Autodesk Inventor part; units mm, degrees
(part 3 of 3)
  line L415 (-154.8147, -40.8229) -> (-168.8197, -40.8229)
  line L416 (-168.8197, -40.8229) -> (-168.8197, -26.8179)
  line L417 (-168.8197, -26.8179) -> (-154.8147, -40.8229) construction
  line L418 (-154.8147, -26.8179) -> (-168.8197, -40.8229) construction
  line L419 (-187.8697, -26.8179) -> (-173.8647, -26.8179)
  line L420 (-173.8647, -26.8179) -> (-173.8647, -40.8229)
  line L421 (-173.8647, -40.8229) -> (-187.8697, -40.8229)
  line L422 (-187.8697, -40.8229) -> (-187.8697, -26.8179)
  line L423 (-187.8697, -26.8179) -> (-173.8647, -40.8229) construction
  line L424 (-173.8647, -26.8179) -> (-187.8697, -40.8229) construction
  line L425 (-214.0317, -26.8179) -> (-200.0267, -26.8179)
  line L426 (-200.0267, -26.8179) -> (-200.0267, -40.8229)
  line L427 (-200.0267, -40.8229) -> (-214.0317, -40.8229)
  line L428 (-214.0317, -40.8229) -> (-214.0317, -26.8179)
  line L429 (-214.0317, -26.8179) -> (-200.0267, -40.8229) construction
  line L430 (-200.0267, -26.8179) -> (-214.0317, -40.8229) construction
  line L431 (-205.1417, -45.8679) -> (-191.1367, -45.8679)
  line L432 (-191.1367, -45.8679) -> (-191.1367, -59.8729)
  line L433 (-191.1367, -59.8729) -> (-205.1417, -59.8729)
  line L434 (-205.1417, -59.8729) -> (-205.1417, -45.8679)
  line L435 (-205.1417, -45.8679) -> (-191.1367, -59.8729) construction
  line L436 (-191.1367, -45.8679) -> (-205.1417, -59.8729) construction
  line L437 (-181.2657, -45.8679) -> (-167.2607, -45.8679)
  line L438 (-167.2607, -45.8679) -> (-167.2607, -59.8729)
  line L439 (-167.2607, -59.8729) -> (-181.2657, -59.8729)
  line L440 (-181.2657, -59.8729) -> (-181.2657, -45.8679)
  line L441 (-181.2657, -45.8679) -> (-167.2607, -59.8729) construction
  line L442 (-167.2607, -45.8679) -> (-181.2657, -59.8729) construction
  line L443 (-83.7297, -45.8679) -> (-69.7247, -45.8679)
  line L444 (-69.7247, -45.8679) -> (-69.7247, -59.8729)
  line L445 (-69.7247, -59.8729) -> (-83.7297, -59.8729)
  line L446 (-83.7297, -59.8729) -> (-83.7297, -45.8679)
  line L447 (-83.7297, -45.8679) -> (-69.7247, -59.8729) construction
  line L448 (-69.7247, -45.8679) -> (-83.7297, -59.8729) construction
  circle A104 centre (-110, -57.5) radius 3.25
  circle A105 centre (0, -57.5) radius 3.25
  line L449 (-143.4772, -45.8679) -> (-143.4772, -58.2679) construction
  line L450 (-9.9772, -45.8679) -> (-9.9772, -58.2679) construction
  line L451 (-219.7432, 11.2821) -> (-213.7432, 11.2821)
  line L452 (-213.7432, 11.2821) -> (-213.7432, -1.1179)
  line L453 (-213.7432, -1.1179) -> (-219.7432, -1.1179)
  line L454 (-219.7432, -1.1179) -> (-219.7432, 11.2821)
  line L455 (-195.7432, 11.2821) -> (-189.7432, 11.2821)
  line L456 (-189.7432, 11.2821) -> (-189.7432, -1.1179)
  line L457 (-189.7432, -1.1179) -> (-195.7432, -1.1179)
  line L458 (-195.7432, -1.1179) -> (-195.7432, 11.2821)
  line L459 (8.4302, -62.3704) -> (-209.6412, -62.3704)
  line L460 (-209.6412, -62.3704) -> (-209.6412, -43.3204)
  line L461 (-209.6412, -43.3204) -> (-223.6412, -43.3204)
  line L462 (-223.6412, -43.3204) -> (-223.6412, 61.3884)
  line L463 (-223.6412, 61.3884) -> (4.4528, 61.3884)
  line L464 (-93, 44) -> (-50, 44)
  line L465 (-50, 44) -> (-50, 37.5)
  line L466 (-50, 37.5) -> (-93, 37.5)
  line L467 (-93, 37.5) -> (-93, 44)
  point P0 (0, 0)
  point P1 (9.3423, 37.558)
  point P2 (-90.4432, 23.3296)
  point P3 (-166.6432, 23.3296)
  point P4 (-190.5192, -14.7704)
  point P5 (-95.2692, -14.7704)
  point P6 (-28.4732, -33.8424)
  point P7 (-85.6172, -33.8204)
  point P8 (-218.2321, -21.7729)
  point P9 (-218.8577, -21.4574)
  dimension "d186" = 0.2
  dimension "d187" = 0.2
  dimension "d188" = 0.2
  dimension "d189" = 0.2
  dimension "d190" = 0.2
  dimension "d191" = 0.2
  dimension "d192" = 0.2
  dimension "d193" = 0.2
  dimension "d194" = 0.2
  dimension "d195" = 0.2
  dimension "d196" = 0.2
  dimension "d198" = 6
  dimension "d199" = 12.4
  dimension "d200" = 6
  dimension "d201" = 14.005
  dimension "d202" = 14.005
  dimension "d203" = 14.005
  dimension "d204" = 14.005
  dimension "d205" = 14.005
  dimension "d206" = 14.005
  dimension "d207" = 14.005
  dimension "d208" = 14.005
  dimension "d209" = 14.005
  dimension "d210" = 14.005
  dimension "d211" = 14.005
  dimension "d212" = 14.005
  dimension "d213" = 14.005
  dimension "d214" = 14.005
  dimension "d215" = 14.005
  dimension "d216" = 14.005
  dimension "d217" = 14.005
  dimension "d218" = 14.005
  dimension "d219" = 14.005
  dimension "d220" = 14.005
  dimension "d221" = 14.005
  dimension "d222" = 14.005
  dimension "d223" = 14.005
  dimension "d224" = 14.005
  dimension "d225" = 14.005
  dimension "d226" = 14.005
  dimension "d227" = 14.005
  dimension "d228" = 14.005
  dimension "d229" = 14.005
  dimension "d230" = 14.005
  dimension "d231" = 14.005
  dimension "d232" = 14.005
  dimension "d233" = 14.005
  dimension "d234" = 14.005
  dimension "d235" = 14.005
  dimension "d236" = 14.005
  dimension "d237" = 14.005
  dimension "d238" = 14.005
  dimension "d239" = 14.005
  dimension "d240" = 14.005
  dimension "d241" = 14.005
  dimension "d242" = 14.005
  dimension "d243" = 14.005
  dimension "d244" = 14.005
  dimension "d245" = 14.005
  dimension "d246" = 14.005
  dimension "d247" = 14.005
  dimension "d248" = 14.005
  dimension "d249" = 14.005
  dimension "d250" = 14.005
  constraints: 776 end point, 128 parallel, 123 midpoint, 72 perpendicular, 63 horizontal, 12 collinear, 10 point on line, 6 centre point, 6 coincident, 5 equal radius, 1 vertical
  measures "d186" distance between parallel lines of L90 L79
  measures "d187" distance from line of point (9.342, 37.558) L80
  measures "d188" distance between parallel lines of L81 L70
  measures "d189" distance between parallel lines of L82 L71
  measures "d190" distance between parallel lines of L83 L72
  measures "d191" distance between parallel lines of L73 L84
  measures "d192" distance between parallel lines of L85 L74
  measures "d193" distance between parallel lines of L86 L75
  measures "d194" distance between parallel lines of L87 L76
  measures "d195" distance between parallel lines of L88 L77
  measures "d196" distance between parallel lines of L89 L78
  measures "d198" distance of L93.start L93.end
  measures "d199" distance of L95.end L93.start
  measures "d200" distance of L97.start L97.end
  measures "d201" distance of L102.end L103.end
  measures "d202" distance of L101.end L102.end
  measures "d203" distance of L108.end L109.end
  measures "d204" distance of L107.end L108.end
  measures "d205" distance of L114.end L115.end
  measures "d206" distance of L113.end L114.end
  measures "d207" distance of L120.end L121.end
  measures "d208" distance of L119.end L120.end
  measures "d209" distance of L126.end L127.end
  measures "d210" distance of L125.end L126.end
  measures "d211" distance of L132.end L133.end
  measures "d212" distance of L131.end L132.end
  measures "d213" distance of L138.end L139.end
  measures "d214" distance of L137.end L138.end
  measures "d215" distance of L144.end L145.end
  measures "d216" distance of L143.end L144.end
  measures "d217" distance of L150.end L151.end
  measures "d218" distance of L149.end L150.end
  measures "d219" distance of L156.end L157.end
  measures "d220" distance of L155.end L156.end
  measures "d221" distance of L162.end L163.end
  measures "d222" distance of L161.end L162.end
  measures "d223" distance of L168.end L169.end
  measures "d224" distance of L167.end L168.end
  measures "d225" distance of L174.end L175.end
  measures "d226" distance of L173.end L174.end
  measures "d227" distance of L180.end L181.end
  measures "d228" distance of L179.end L180.end
  measures "d229" distance of L186.end L187.end
  measures "d230" distance of L185.end L186.end
  measures "d231" distance of L192.end L193.end
  measures "d232" distance of L191.end L192.end
  measures "d233" distance of L198.end L199.end
  measures "d234" distance of L197.end L198.end
  measures "d235" distance of L204.end L205.end
  measures "d236" distance of L203.end L204.end
  measures "d237" distance of L210.end L211.end
  measures "d238" distance of L209.end L210.end
  measures "d239" distance of L216.end L217.end
  measures "d240" distance of L215.end L216.end
  measures "d241" distance of L222.end L223.end
  measures "d242" distance of L221.end L222.end
  measures "d243" distance of L228.end L229.end
  measures "d244" distance of L227.end L228.end
  measures "d245" distance of L234.end L235.end
  measures "d246" distance of L233.end L234.end
  measures "d247" distance of L240.end L241.end
  measures "d248" distance of L239.end L240.end
  measures "d249" distance of L246.end L247.end
  measures "d250" distance of L245.end L246.end
extrude "Thin Plate" add sketch "Sketch5" along normal blind 0.25
sketch "Sketch7" plane through (0, 0, 0.25) normal (0, 0, 1) x (1, 0, 0)
  line L0 (-76.4012, 61.3884) -> (-76.4012, 42.3884) construction
  line L1 (-76.4012, 42.3884) -> (-194.4012, 42.3884) construction
  line L2 (-93, 44) -> (-50, 44) construction
  line L3 (-93, 37.5) -> (-93, 44) construction
  line L4 (-66.3852, 42.3884) -> (-66.3852, 61.3884) construction
  line L5 (51.6148, 42.3884) -> (-66.3852, 42.3884) construction
  line L6 (-50, 44) -> (-50, 37.5) construction
  line L7 (-204.6412, 61.3884) -> (-204.6412, 42.3884) construction
  line L8 (-204.6412, 42.3884) -> (-223.6412, 42.3884) construction
  line L9 (71.4568, 32.8296) -> (-223.6412, 32.8296) construction
  line L10 (14.2318, 13.9046) -> (14.2318, 37.558) construction
  line L11 (4.4528, 13.9046) -> (14.2318, 13.9046) projected
  line L12 (4.4528, -5.3455) -> (4.4528, 13.9046) projected
  line L13 (9.6598, -5.3455) -> (4.4528, -5.3455) projected
  line L14 (9.6598, -24.1954) -> (9.6598, -5.3455) projected
  line L15 (0.0048, -24.1954) -> (9.6598, -24.1954) projected
  line L16 (0.0048, -49.2614) -> (0.0048, -24.1954) projected
  line L17 (8.4302, -49.2614) -> (0.0048, -49.2614) projected
  line L18 (8.4302, -62.3704) -> (8.4302, -49.2614) projected
  line L19 (-209.6412, -62.3704) -> (8.4302, -62.3704) construction
  line L20 (-209.6412, -43.3204) -> (-209.6412, -62.3704) projected
  line L21 (8.4302, -62.3704) -> (-209.6412, -62.3704)
  line L22 (-223.6412, -43.3204) -> (-209.6412, -43.3204) projected
  line L23 (-223.6412, 61.3884) -> (-223.6412, -43.3204) construction
  line L24 (-223.6412, -43.3204) -> (-223.6412, 32.8296)
  line L25 (-223.6412, 61.3884) -> (-223.6412, -43.3204) projected
  line L26 (-223.6412, 32.8296) -> (14.2318, 32.8296)
  line L27 (14.2318, 32.8296) -> (14.2318, 13.9046)
  line L28 (4.4528, 37.558) -> (4.4528, 61.3884) construction
  line L29 (4.4528, 61.3884) -> (-223.6412, 61.3884) construction
  line L30 (-194.4012, 42.3884) -> (-194.4012, 61.3884) construction
  line L31 (-223.6412, 42.3884) -> (-223.6412, 61.3884)
  line L32 (-223.6412, 61.3884) -> (-204.6412, 61.3884)
  line L33 (-204.6412, 61.3884) -> (-204.6412, 42.3884)
  line L34 (-204.6412, 42.3884) -> (-223.6412, 42.3884)
  line L35 (-194.4012, 42.3884) -> (-194.4012, 61.3884)
  line L36 (-194.4012, 61.3884) -> (-76.4012, 61.3884)
  line L37 (-76.4012, 61.3884) -> (-76.4012, 44)
  line L38 (-76.4012, 44) -> (-93, 44)
  line L39 (-93, 44) -> (-93, 42.3884)
  line L40 (-93, 37.5) -> (-93, 44) projected
  line L41 (-93, 42.3884) -> (-194.4012, 42.3884)
  line L42 (-66.3852, 61.3884) -> (-66.3852, 44)
  line L43 (-66.3852, 44) -> (-50, 44)
  line L44 (-50, 44) -> (-50, 42.3884)
  line L45 (-50, 42.3884) -> (4.4528, 42.3884)
  line L46 (4.4528, 42.3884) -> (4.4528, 61.3884)
  line L47 (4.4528, 61.3884) -> (-66.3852, 61.3884)
  line L48 (0.0048, -49.2614) -> (0.0048, -24.1954) projected
  line L49 (0.0048, -24.1954) -> (9.6598, -24.1954) projected
  line L50 (9.6598, -24.1954) -> (9.6598, -5.3455) projected
  line L51 (9.6598, -5.3455) -> (4.4528, -5.3455) projected
  line L52 (4.4528, -5.3455) -> (4.4528, 13.9046) projected
  line L53 (4.4528, 13.9046) -> (14.2318, 13.9046) projected
  line L54 (14.2318, 13.9046) -> (14.2318, 37.558) projected
  line L55 (14.2318, 37.558) -> (4.4528, 37.558) projected
  line L56 (4.4528, 37.558) -> (4.4528, 61.3884) projected
  line L57 (4.4528, 61.3884) -> (-223.6412, 61.3884) projected
  line L58 (-223.6412, 61.3884) -> (-223.6412, -43.3204) projected
  line L59 (-223.6412, -43.3204) -> (-209.6412, -43.3204) projected
  line L60 (-209.6412, -43.3204) -> (-209.6412, -62.3704) projected
  line L61 (-209.6412, -62.3704) -> (8.4302, -62.3704) projected
  line L62 (8.4302, -62.3704) -> (8.4302, -49.2614) projected
  line L63 (8.4302, -49.2614) -> (0.0048, -49.2614) projected
  circle A0 centre (0, -57.5) radius 3.25 projected
  circle A1 centre (-110, -57.5) radius 3.25 projected
  circle A2 centre (0, 37.6384) radius 3.25 projected
  circle A3 centre (-110, 37.6384) radius 3.25 projected
  circle A4 centre (-220, 37.6384) radius 3.25 projected
  line L64 (-93, 44) -> (-50, 44) projected
  line L65 (-50, 44) -> (-50, 37.5) projected
  line L66 (-50, 37.5) -> (-93, 37.5) projected
  line L67 (-93, 37.5) -> (-93, 44) projected
  line L68 (-195.7432, 11.2821) -> (-189.7432, 11.2821) projected
  line L69 (-189.7432, 11.2821) -> (-189.7432, -1.1179) projected
  line L70 (-189.7432, -1.1179) -> (-195.7432, -1.1179) projected
  line L71 (-195.7432, -1.1179) -> (-195.7432, 11.2821) projected
  line L72 (-219.7432, 11.2821) -> (-213.7432, 11.2821) projected
  line L73 (-213.7432, 11.2821) -> (-213.7432, -1.1179) projected
  line L74 (-213.7432, -1.1179) -> (-219.7432, -1.1179) projected
  line L75 (-219.7432, -1.1179) -> (-219.7432, 11.2821) projected
  line L76 (-83.7297, -45.8679) -> (-69.7247, -45.8679) projected
  line L77 (-69.7247, -45.8679) -> (-69.7247, -59.8729) projected
  line L78 (-69.7247, -59.8729) -> (-83.7297, -59.8729) projected
  line L79 (-83.7297, -59.8729) -> (-83.7297, -45.8679) projected
  line L80 (-181.2657, -45.8679) -> (-167.2607, -45.8679) projected
  line L81 (-167.2607, -45.8679) -> (-167.2607, -59.8729) projected
  line L82 (-167.2607, -59.8729) -> (-181.2657, -59.8729) projected
  line L83 (-181.2657, -59.8729) -> (-181.2657, -45.8679) projected
  line L84 (-205.1417, -45.8679) -> (-191.1367, -45.8679) projected
  line L85 (-191.1367, -45.8679) -> (-191.1367, -59.8729) projected
  line L86 (-191.1367, -59.8729) -> (-205.1417, -59.8729) projected
  line L87 (-205.1417, -59.8729) -> (-205.1417, -45.8679) projected
  line L88 (-214.0317, -26.8179) -> (-200.0267, -26.8179) projected
  line L89 (-200.0267, -26.8179) -> (-200.0267, -40.8229) projected
  line L90 (-200.0267, -40.8229) -> (-214.0317, -40.8229) projected
  line L91 (-214.0317, -40.8229) -> (-214.0317, -26.8179) projected
  line L92 (-187.8697, -26.8179) -> (-173.8647, -26.8179) projected
  line L93 (-173.8647, -26.8179) -> (-173.8647, -40.8229) projected
  line L94 (-173.8647, -40.8229) -> (-187.8697, -40.8229) projected
  line L95 (-187.8697, -40.8229) -> (-187.8697, -26.8179) projected
  line L96 (-168.8197, -26.8179) -> (-154.8147, -26.8179) projected
  line L97 (-154.8147, -26.8179) -> (-154.8147, -40.8229) projected
  line L98 (-154.8147, -40.8229) -> (-168.8197, -40.8229) projected
  line L99 (-168.8197, -40.8229) -> (-168.8197, -26.8179) projected
  line L100 (-149.7697, -26.8179) -> (-135.7647, -26.8179) projected
  line L101 (-135.7647, -26.8179) -> (-135.7647, -40.8229) projected
  line L102 (-135.7647, -40.8229) -> (-149.7697, -40.8229) projected
  line L103 (-149.7697, -40.8229) -> (-149.7697, -26.8179) projected
  line L104 (-130.7197, -26.8179) -> (-116.7147, -26.8179) projected
  line L105 (-116.7147, -26.8179) -> (-116.7147, -40.8229) projected
  line L106 (-116.7147, -40.8229) -> (-130.7197, -40.8229) projected
  line L107 (-130.7197, -40.8229) -> (-130.7197, -26.8179) projected
  line L108 (-111.6697, -26.8179) -> (-97.6647, -26.8179) projected
  line L109 (-97.6647, -26.8179) -> (-97.6647, -40.8229) projected
  line L110 (-97.6647, -40.8229) -> (-111.6697, -40.8229) projected
  line L111 (-111.6697, -40.8229) -> (-111.6697, -26.8179) projected
  line L112 (-92.6197, -26.8179) -> (-78.6147, -26.8179) projected
  line L113 (-78.6147, -26.8179) -> (-78.6147, -40.8229) projected
  line L114 (-78.6147, -40.8229) -> (-92.6197, -40.8229) projected
  line L115 (-92.6197, -40.8229) -> (-92.6197, -26.8179) projected
  line L116 (-73.5697, -26.8179) -> (-59.5647, -26.8179) projected
  line L117 (-59.5647, -26.8179) -> (-59.5647, -40.8229) projected
  line L118 (-59.5647, -40.8229) -> (-73.5697, -40.8229) projected
  line L119 (-73.5697, -40.8229) -> (-73.5697, -26.8179) projected
  line L120 (-54.5197, -26.8179) -> (-40.5147, -26.8179) projected
  line L121 (-40.5147, -26.8179) -> (-40.5147, -40.8229) projected
  line L122 (-40.5147, -40.8229) -> (-54.5197, -40.8229) projected
  line L123 (-54.5197, -40.8229) -> (-54.5197, -26.8179) projected
  line L124 (-35.4757, -26.8399) -> (-21.4707, -26.8399) projected
  line L125 (-21.4707, -26.8399) -> (-21.4707, -40.8449) projected
  line L126 (-21.4707, -40.8449) -> (-35.4757, -40.8449) projected
  line L127 (-35.4757, -40.8449) -> (-35.4757, -26.8399) projected
  line L128 (-16.4257, -26.8399) -> (-2.4207, -26.8399) projected
  line L129 (-2.4207, -26.8399) -> (-2.4207, -40.8449) projected
  line L130 (-2.4207, -40.8449) -> (-16.4257, -40.8449) projected
  line L131 (-16.4257, -40.8449) -> (-16.4257, -26.8399) projected
  line L132 (-6.7677, -7.7679) -> (7.2373, -7.7679) projected
  line L133 (7.2373, -7.7679) -> (7.2373, -21.7729) projected
  line L134 (7.2373, -21.7729) -> (-6.7677, -21.7729) projected
  line L135 (-6.7677, -21.7729) -> (-6.7677, -7.7679) projected
  line L136 (-26.0717, -7.7679) -> (-12.0667, -7.7679) projected
  line L137 (-12.0667, -7.7679) -> (-12.0667, -21.7729) projected
  line L138 (-12.0667, -21.7729) -> (-26.0717, -21.7729) projected
  line L139 (-26.0717, -21.7729) -> (-26.0717, -7.7679) projected
  line L140 (-45.1217, -7.7679) -> (-31.1167, -7.7679) projected
  line L141 (-31.1167, -7.7679) -> (-31.1167, -21.7729) projected
  line L142 (-31.1167, -21.7729) -> (-45.1217, -21.7729) projected
  line L143 (-45.1217, -21.7729) -> (-45.1217, -7.7679) projected
  line L144 (-64.1717, -7.7679) -> (-50.1667, -7.7679) projected
  line L145 (-50.1667, -7.7679) -> (-50.1667, -21.7729) projected
  line L146 (-50.1667, -21.7729) -> (-64.1717, -21.7729) projected
  line L147 (-64.1717, -21.7729) -> (-64.1717, -7.7679) projected
  line L148 (-83.2217, -7.7679) -> (-69.2167, -7.7679) projected
  line L149 (-69.2167, -7.7679) -> (-69.2167, -21.7729) projected
  line L150 (-69.2167, -21.7729) -> (-83.2217, -21.7729) projected
  line L151 (-83.2217, -21.7729) -> (-83.2217, -7.7679) projected
  line L152 (-102.2717, -7.7679) -> (-88.2667, -7.7679) projected
  line L153 (-88.2667, -7.7679) -> (-88.2667, -21.7729) projected
  line L154 (-88.2667, -21.7729) -> (-102.2717, -21.7729) projected
  line L155 (-102.2717, -21.7729) -> (-102.2717, -7.7679) projected
  line L156 (-121.3217, -7.7679) -> (-107.3167, -7.7679) projected
  line L157 (-107.3167, -7.7679) -> (-107.3167, -21.7729) projected
  line L158 (-107.3167, -21.7729) -> (-121.3217, -21.7729) projected
  line L159 (-121.3217, -21.7729) -> (-121.3217, -7.7679) projected
  line L160 (-140.3717, -7.7679) -> (-126.3667, -7.7679) projected
  line L161 (-126.3667, -7.7679) -> (-126.3667, -21.7729) projected
  line L162 (-126.3667, -21.7729) -> (-140.3717, -21.7729) projected
  line L163 (-140.3717, -21.7729) -> (-140.3717, -7.7679) projected
  line L164 (-159.4217, -7.7679) -> (-145.4167, -7.7679) projected
  line L165 (-145.4167, -7.7679) -> (-145.4167, -21.7729) projected
  line L166 (-145.4167, -21.7729) -> (-159.4217, -21.7729) projected
  line L167 (-159.4217, -21.7729) -> (-159.4217, -7.7679) projected
  line L168 (-178.4717, -7.7679) -> (-164.4667, -7.7679) projected
  line L169 (-164.4667, -7.7679) -> (-164.4667, -21.7729) projected
  line L170 (-164.4667, -21.7729) -> (-178.4717, -21.7729) projected
  line L171 (-178.4717, -21.7729) -> (-178.4717, -7.7679) projected
  line L172 (-197.5217, -7.7679) -> (-183.5167, -7.7679) projected
  line L173 (-183.5167, -7.7679) -> (-183.5167, -21.7729) projected
  line L174 (-183.5167, -21.7729) -> (-197.5217, -21.7729) projected
  line L175 (-197.5217, -21.7729) -> (-197.5217, -7.7679) projected
  line L176 (-211.7457, 11.2821) -> (-197.7407, 11.2821) projected
  line L177 (-197.7407, 11.2821) -> (-197.7407, -2.7229) projected
  line L178 (-197.7407, -2.7229) -> (-211.7457, -2.7229) projected
  line L179 (-211.7457, -2.7229) -> (-211.7457, 11.2821) projected
  line L180 (-183.2977, 11.2821) -> (-169.2927, 11.2821) projected
  line L181 (-169.2927, 11.2821) -> (-169.2927, -2.7229) projected
  line L182 (-169.2927, -2.7229) -> (-183.2977, -2.7229) projected
  line L183 (-183.2977, -2.7229) -> (-183.2977, 11.2821) projected
  line L184 (-164.2477, 11.2821) -> (-150.2427, 11.2821) projected
  line L185 (-150.2427, 11.2821) -> (-150.2427, -2.7229) projected
  line L186 (-150.2427, -2.7229) -> (-164.2477, -2.7229) projected
  line L187 (-164.2477, -2.7229) -> (-164.2477, 11.2821) projected
  line L188 (-145.1977, 11.2821) -> (-131.1927, 11.2821) projected
  line L189 (-131.1927, 11.2821) -> (-131.1927, -2.7229) projected
  line L190 (-131.1927, -2.7229) -> (-145.1977, -2.7229) projected
  line L191 (-145.1977, -2.7229) -> (-145.1977, 11.2821) projected
  line L192 (-112.1427, 11.2821) -> (-112.1427, -2.7229) projected
  line L193 (-112.1427, -2.7229) -> (-126.1477, -2.7229) projected
  line L194 (-126.1477, -2.7229) -> (-126.1477, 11.2821) projected
  line L195 (-126.1477, 11.2821) -> (-112.1427, 11.2821) projected
  line L196 (-107.0977, 11.2033) -> (-93.0927, 11.2033) projected
  line L197 (-93.0927, 11.2033) -> (-93.0927, -2.8017) projected
  line L198 (-93.0927, -2.8017) -> (-107.0977, -2.8017) projected
  line L199 (-107.0977, -2.8017) -> (-107.0977, 11.2033) projected
  line L200 (-88.0477, 11.2821) -> (-74.0427, 11.2821) projected
  line L201 (-74.0427, 11.2821) -> (-74.0427, -2.7229) projected
  line L202 (-74.0427, -2.7229) -> (-88.0477, -2.7229) projected
  line L203 (-88.0477, -2.7229) -> (-88.0477, 11.2821) projected
  line L204 (-68.9977, 11.2821) -> (-54.9927, 11.2821) projected
  line L205 (-54.9927, 11.2821) -> (-54.9927, -2.7229) projected
  line L206 (-54.9927, -2.7229) -> (-68.9977, -2.7229) projected
  line L207 (-68.9977, -2.7229) -> (-68.9977, 11.2821) projected
  line L208 (-49.9477, 11.2821) -> (-35.9427, 11.2821) projected
  line L209 (-35.9427, 11.2821) -> (-35.9427, -2.7229) projected
  line L210 (-35.9427, -2.7229) -> (-49.9477, -2.7229) projected
  line L211 (-49.9477, -2.7229) -> (-49.9477, 11.2821) projected
  line L212 (-30.8977, 11.2821) -> (-16.8927, 11.2821) projected
  line L213 (-16.8927, 11.2821) -> (-16.8927, -2.7229) projected
  line L214 (-16.8927, -2.7229) -> (-30.8977, -2.7229) projected
  line L215 (-30.8977, -2.7229) -> (-30.8977, 11.2821) projected
  line L216 (-11.8477, 11.2821) -> (2.1573, 11.2821) projected
  line L217 (2.1573, 11.2821) -> (2.1573, -2.7229) projected
  line L218 (2.1573, -2.7229) -> (-11.8477, -2.7229) projected
  line L219 (-11.8477, -2.7229) -> (-11.8477, 11.2821) projected
  line L220 (-2.1957, 30.3321) -> (11.8093, 30.3321) projected
  line L221 (11.8093, 30.3321) -> (11.8093, 16.3271) projected
  line L222 (11.8093, 16.3271) -> (-2.1957, 16.3271) projected
  line L223 (-2.1957, 16.3271) -> (-2.1957, 30.3321) projected
  line L224 (-21.2457, 30.3321) -> (-7.2407, 30.3321) projected
  line L225 (-7.2407, 30.3321) -> (-7.2407, 16.3271) projected
  line L226 (-7.2407, 16.3271) -> (-21.2457, 16.3271) projected
  line L227 (-21.2457, 16.3271) -> (-21.2457, 30.3321) projected
  line L228 (-40.2957, 30.3321) -> (-26.2907, 30.3321) projected
  line L229 (-26.2907, 30.3321) -> (-26.2907, 16.3271) projected
  line L230 (-26.2907, 16.3271) -> (-40.2957, 16.3271) projected
  line L231 (-40.2957, 16.3271) -> (-40.2957, 30.3321) projected
  line L232 (-59.3457, 30.3321) -> (-45.3407, 30.3321) projected
  line L233 (-45.3407, 30.3321) -> (-45.3407, 16.3271) projected
  line L234 (-45.3407, 16.3271) -> (-59.3457, 16.3271) projected
  line L235 (-59.3457, 16.3271) -> (-59.3457, 30.3321) projected
  line L236 (-78.3957, 30.3321) -> (-64.3907, 30.3321) projected
  line L237 (-64.3907, 30.3321) -> (-64.3907, 16.3271) projected
  line L238 (-64.3907, 16.3271) -> (-78.3957, 16.3271) projected
  line L239 (-78.3957, 16.3271) -> (-78.3957, 30.3321) projected
  line L240 (-173.6457, 30.3321) -> (-159.6407, 30.3321) projected
  line L241 (-159.6407, 30.3321) -> (-159.6407, 16.3271) projected
  line L242 (-159.6407, 16.3271) -> (-173.6457, 16.3271) projected
  line L243 (-173.6457, 16.3271) -> (-173.6457, 30.3321) projected
  line L244 (-97.4457, 30.3321) -> (-83.4407, 30.3321) projected
  line L245 (-83.4407, 30.3321) -> (-83.4407, 16.3271) projected
  line L246 (-83.4407, 16.3271) -> (-97.4457, 16.3271) projected
  line L247 (-97.4457, 16.3271) -> (-97.4457, 30.3321) projected
  line L248 (-116.4957, 30.3321) -> (-102.4907, 30.3321) projected
  line L249 (-102.4907, 30.3321) -> (-102.4907, 16.3271) projected
  line L250 (-102.4907, 16.3271) -> (-116.4957, 16.3271) projected
  line L251 (-116.4957, 16.3271) -> (-116.4957, 30.3321) projected
  line L252 (-135.5457, 30.3321) -> (-121.5407, 30.3321) projected
  line L253 (-121.5407, 30.3321) -> (-121.5407, 16.3271) projected
  line L254 (-121.5407, 16.3271) -> (-135.5457, 16.3271) projected
  line L255 (-135.5457, 16.3271) -> (-135.5457, 30.3321) projected
  line L256 (-154.5957, 30.3321) -> (-140.5907, 30.3321) projected
  line L257 (-140.5907, 30.3321) -> (-140.5907, 16.3271) projected
  line L258 (-140.5907, 16.3271) -> (-154.5957, 16.3271) projected
  line L259 (-154.5957, 16.3271) -> (-154.5957, 30.3321) projected
  line L260 (-192.6957, 30.3321) -> (-178.6907, 30.3321) projected
  line L261 (-178.6907, 30.3321) -> (-178.6907, 16.3271) projected
  line L262 (-178.6907, 16.3271) -> (-192.6957, 16.3271) projected
  line L263 (-192.6957, 16.3271) -> (-192.6957, 30.3321) projected
  line L264 (-216.4737, 30.3321) -> (-202.4687, 30.3321) projected
  line L265 (-202.4687, 30.3321) -> (-202.4687, 16.3271) projected
  line L266 (-202.4687, 16.3271) -> (-216.4737, 16.3271) projected
  line L267 (-216.4737, 16.3271) -> (-216.4737, 30.3321) projected
  line L268 (-14.3877, 58.9889) -> (-0.3827, 58.9889) projected
  line L269 (-0.3827, 58.9889) -> (-0.3827, 44.9839) projected
  line L270 (-0.3827, 44.9839) -> (-14.3877, 44.9839) projected
  line L271 (-14.3877, 44.9839) -> (-14.3877, 58.9889) projected
  line L272 (-38.2637, 58.9889) -> (-24.2587, 58.9889) projected
  line L273 (-24.2587, 58.9889) -> (-24.2587, 44.9839) projected
  line L274 (-24.2587, 44.9839) -> (-38.2637, 44.9839) projected
  line L275 (-38.2637, 44.9839) -> (-38.2637, 58.9889) projected
  line L276 (-62.1457, 58.9889) -> (-48.1407, 58.9889) projected
  line L277 (-48.1407, 58.9889) -> (-48.1407, 44.9839) projected
  line L278 (-48.1407, 44.9839) -> (-62.1457, 44.9839) projected
  line L279 (-62.1457, 44.9839) -> (-62.1457, 58.9889) projected
  line L280 (-94.6517, 58.9889) -> (-80.6467, 58.9889) projected
  line L281 (-80.6467, 58.9889) -> (-80.6467, 44.9839) projected
  line L282 (-80.6467, 44.9839) -> (-94.6517, 44.9839) projected
  line L283 (-94.6517, 44.9839) -> (-94.6517, 58.9889) projected
  line L284 (-118.5277, 58.9889) -> (-104.5227, 58.9889) projected
  line L285 (-104.5227, 58.9889) -> (-104.5227, 44.9839) projected
  line L286 (-104.5227, 44.9839) -> (-118.5277, 44.9839) projected
  line L287 (-118.5277, 44.9839) -> (-118.5277, 58.9889) projected
  line L288 (-142.4037, 58.9609) -> (-128.3987, 58.9609) projected
  line L289 (-128.3987, 58.9609) -> (-128.3987, 44.9559) projected
  line L290 (-128.3987, 44.9559) -> (-142.4037, 44.9559) projected
  line L291 (-142.4037, 44.9559) -> (-142.4037, 58.9609) projected
  line L292 (-166.2797, 58.9889) -> (-152.2747, 58.9889) projected
  line L293 (-152.2747, 58.9889) -> (-152.2747, 44.9839) projected
  line L294 (-152.2747, 44.9839) -> (-166.2797, 44.9839) projected
  line L295 (-166.2797, 44.9839) -> (-166.2797, 58.9889) projected
  line L296 (-190.0953, 59.1041) -> (-176.0903, 59.1041) projected
  line L297 (-176.0903, 59.1041) -> (-176.0903, 45.0991) projected
  line L298 (-176.0903, 45.0991) -> (-190.0953, 45.0991) projected
  line L299 (-190.0953, 45.0991) -> (-190.0953, 59.1041) projected
  line L300 (-221.1437, 58.8909) -> (-207.1387, 58.8909) projected
  line L301 (-207.1387, 58.8909) -> (-207.1387, 44.8859) projected
  line L302 (-207.1387, 44.8859) -> (-221.1437, 44.8859) projected
  line L303 (-221.1437, 44.8859) -> (-221.1437, 58.8909) projected
  line L304 (-12.9772, -45.8679) -> (-6.9772, -45.8679) projected
  line L305 (-6.9772, -45.8679) -> (-6.9772, -58.2679) projected
  line L306 (-6.9772, -58.2679) -> (-12.9772, -58.2679) projected
  line L307 (-12.9772, -58.2679) -> (-12.9772, -45.8679) projected
  line L308 (-146.4772, -45.8679) -> (-140.4772, -45.8679) projected
  line L309 (-140.4772, -45.8679) -> (-140.4772, -58.2679) projected
  line L310 (-140.4772, -58.2679) -> (-146.4772, -58.2679) projected
  line L311 (-146.4772, -58.2679) -> (-146.4772, -45.8679) projected
  line L312 (-204.8527, -7.7679) -> (-204.8527, -21.7729) projected
  line L313 (-204.8527, -21.7729) -> (-218.2321, -21.7729) projected
  arc A5 (-218.8577, -21.4574) -> (-218.2321, -21.7729) centre (-220, -24.5) ccw projected
  line L314 (-218.8577, -21.4574) -> (-218.8577, -7.7679) projected
  line L315 (-218.8577, -7.7679) -> (-204.8527, -7.7679) projected
  point P0 (0, 0)
  constraints: 40 end point, 12 point on line, 9 collinear, 5 perpendicular
extrude "Switch Supports" add sketch "Sketch7" along normal blind 3 contours L12 L13 L14 L15 L16 L17 L18 L21 L20 L22 L24 L26 L27 L11 | L25 L32 L33 L34 | L45 L44 L43 L42 L47 L46 | L36 L37 L38 L39 L41 L35
sketch "Sketch8" plane through (0, 0, 0) normal (0, 0, -1) x (-1, 0, 0)
  line L0 (6.9772, -42.3679) -> (12.9772, -42.3679)
  line L1 (12.9772, -48.3679) -> (12.9772, -60.2679)
  line L2 (12.9772, -60.2679) -> (6.9772, -60.2679)
  line L3 (6.9772, -60.2679) -> (6.9772, -42.3679)
  line L4 (140.4772, -42.3679) -> (146.4772, -42.3679)
  line L5 (146.4772, -42.3679) -> (146.4772, -60.2679)
  line L6 (146.4772, -60.2679) -> (140.4772, -60.2679)
  line L7 (140.4772, -60.2679) -> (140.4772, -48.3679)
  line L8 (12.9772, -45.8679) -> (6.9772, -45.8679) projected
  line L9 (6.9772, -58.2679) -> (12.9772, -58.2679) projected
  line L10 (12.9772, -58.2679) -> (12.9772, -45.8679) projected
  line L11 (6.9772, -45.8679) -> (6.9772, -58.2679) projected
  line L12 (140.4772, -45.8679) -> (140.4772, -58.2679) projected
  line L13 (146.4772, -58.2679) -> (146.4772, -45.8679) projected
  line L14 (12.9772, -42.3679) -> (140.4772, -42.3679)
  line L15 (12.9772, -48.3679) -> (140.4772, -48.3679)
  line L16 (195.7432, -1.1179) -> (189.7432, -1.1179)
  line L17 (213.7432, 14.7821) -> (219.7432, 14.7821)
  line L18 (219.7432, 14.7821) -> (219.7432, -3.1179)
  line L19 (219.7432, -3.1179) -> (213.7432, -3.1179)
  line L20 (213.7432, -3.1179) -> (213.7432, 8.7821)
  line L21 (189.7432, 14.7821) -> (195.7432, 14.7821)
  line L22 (195.7432, 8.7821) -> (195.7432, -3.1179)
  line L23 (195.7432, -3.1179) -> (189.7432, -3.1179)
  line L24 (189.7432, -3.1179) -> (189.7432, 14.7821)
  line L25 (195.7432, 11.2821) -> (189.7432, 11.2821) projected
  line L26 (189.7432, 11.2821) -> (189.7432, -1.1179) projected
  line L27 (195.7432, -1.1179) -> (195.7432, 11.2821) projected
  line L28 (213.7432, 11.2821) -> (213.7432, -1.1179) projected
  line L29 (219.7432, -1.1179) -> (219.7432, 11.2821) projected
  line L30 (195.7432, 14.7821) -> (213.7432, 14.7821)
  line L31 (195.7432, 8.7821) -> (213.7432, 8.7821)
  point P0 (0, 0)
  dimension "d339" = 3.5
  dimension "d340" = 2
  dimension "d341" = 6
  dimension "d342" = 3.5
  dimension "d343" = 2
  dimension "d344" = 6
  constraints: 42 end point, 12 collinear, 8 parallel, 6 horizontal, 6 perpendicular, 4 point on line
  measures "d339" distance between parallel lines of L0 L8
  measures "d340" distance between parallel lines of L2 L9
  measures "d341" distance between parallel lines of L15 L14
  measures "d342" distance between parallel lines of L21 L25
  measures "d343" distance between parallel lines of L23 L16
  measures "d344" distance between parallel lines of L31 L30
extrude "Stabilizer cuts" cut sketch "Sketch8" against normal blind 2
sketch "Sketch9" plane through (0, 0, 3.25) normal (0, 0, 1) x (1, 0, 0)
  line L0 (14.2318, 32.8296) -> (-223.6412, 32.8296) construction
  line L1 (-223.6412, 32.8296) -> (-223.6412, -43.3204) construction
  line L2 (-223.6412, -43.3204) -> (-209.6412, -43.3204) construction
  line L3 (-209.6412, -43.3204) -> (-209.6412, -62.3704) construction
  line L4 (-209.6412, -62.3704) -> (8.4302, -62.3704) construction
  line L5 (8.4302, -62.3704) -> (8.4302, -49.2614) construction
  line L6 (8.4302, -49.2614) -> (0.0048, -49.2614) construction
  line L7 (0.0048, -49.2614) -> (0.0048, -24.1954) construction
  line L8 (0.0048, -24.1954) -> (9.6598, -24.1954) construction
  line L9 (9.6598, -24.1954) -> (9.6598, -5.3455) construction
  line L10 (9.6598, -5.3455) -> (4.4528, -5.3455) construction
  line L11 (4.4528, -5.3455) -> (4.4528, 13.9046) construction
  line L12 (4.4528, 13.9046) -> (14.2318, 13.9046) construction
  line L13 (14.2318, 13.9046) -> (14.2318, 32.8296) construction
  circle A0 centre (0, -57.5) radius 3.25 construction
  circle A1 centre (-110, -57.5) radius 3.25 construction
  line L14 (-218.8577, -21.4574) -> (-218.8577, -7.7679) construction
  line L15 (-218.8577, -7.7679) -> (-204.8527, -7.7679) construction
  line L16 (-204.8527, -7.7679) -> (-204.8527, -21.7729) construction
  line L17 (-204.8527, -21.7729) -> (-218.2321, -21.7729) construction
  arc A2 (-218.8577, -21.4574) -> (-218.2321, -21.7729) centre (-220, -24.5) ccw construction
  line L18 (-146.4772, -45.8679) -> (-140.4772, -45.8679) construction
  line L19 (-140.4772, -45.8679) -> (-140.4772, -58.2679) construction
  line L20 (-140.4772, -58.2679) -> (-146.4772, -58.2679) construction
  line L21 (-146.4772, -58.2679) -> (-146.4772, -45.8679) construction
  line L22 (-12.9772, -45.8679) -> (-6.9772, -45.8679) construction
  line L23 (-6.9772, -45.8679) -> (-6.9772, -58.2679) construction
  line L24 (-6.9772, -58.2679) -> (-12.9772, -58.2679) construction
  line L25 (-12.9772, -58.2679) -> (-12.9772, -45.8679) construction
  line L26 (-216.4737, 30.3321) -> (-202.4687, 30.3321) construction
  line L27 (-202.4687, 30.3321) -> (-202.4687, 16.3271) construction
  line L28 (-202.4687, 16.3271) -> (-216.4737, 16.3271) construction
  line L29 (-216.4737, 16.3271) -> (-216.4737, 30.3321) construction
  line L30 (-192.6957, 30.3321) -> (-178.6907, 30.3321) construction
  line L31 (-178.6907, 30.3321) -> (-178.6907, 16.3271) construction
  line L32 (-178.6907, 16.3271) -> (-192.6957, 16.3271) construction
  line L33 (-192.6957, 16.3271) -> (-192.6957, 30.3321) construction
  line L34 (-154.5957, 30.3321) -> (-140.5907, 30.3321) construction
  line L35 (-140.5907, 30.3321) -> (-140.5907, 16.3271) construction
  line L36 (-140.5907, 16.3271) -> (-154.5957, 16.3271) construction
  line L37 (-154.5957, 16.3271) -> (-154.5957, 30.3321) construction
  line L38 (-135.5457, 30.3321) -> (-121.5407, 30.3321) construction
  line L39 (-121.5407, 30.3321) -> (-121.5407, 16.3271) construction
  line L40 (-121.5407, 16.3271) -> (-135.5457, 16.3271) construction
  line L41 (-135.5457, 16.3271) -> (-135.5457, 30.3321) construction
  line L42 (-116.4957, 30.3321) -> (-102.4907, 30.3321) construction
  line L43 (-102.4907, 30.3321) -> (-102.4907, 16.3271) construction
  line L44 (-102.4907, 16.3271) -> (-116.4957, 16.3271) construction
  line L45 (-116.4957, 16.3271) -> (-116.4957, 30.3321) construction
  line L46 (-97.4457, 30.3321) -> (-83.4407, 30.3321) construction
  line L47 (-83.4407, 30.3321) -> (-83.4407, 16.3271) construction
  line L48 (-83.4407, 16.3271) -> (-97.4457, 16.3271) construction
  line L49 (-97.4457, 16.3271) -> (-97.4457, 30.3321) construction
  line L50 (-173.6457, 30.3321) -> (-159.6407, 30.3321) construction
  line L51 (-159.6407, 30.3321) -> (-159.6407, 16.3271) construction
  line L52 (-159.6407, 16.3271) -> (-173.6457, 16.3271) construction
  line L53 (-173.6457, 16.3271) -> (-173.6457, 30.3321) construction
  line L54 (-78.3957, 30.3321) -> (-64.3907, 30.3321) construction
  line L55 (-64.3907, 30.3321) -> (-64.3907, 16.3271) construction
  line L56 (-64.3907, 16.3271) -> (-78.3957, 16.3271) construction
  line L57 (-78.3957, 16.3271) -> (-78.3957, 30.3321) construction
  line L58 (-59.3457, 30.3321) -> (-45.3407, 30.3321) construction
  line L59 (-45.3407, 30.3321) -> (-45.3407, 16.3271) construction
  line L60 (-45.3407, 16.3271) -> (-59.3457, 16.3271) construction
  line L61 (-59.3457, 16.3271) -> (-59.3457, 30.3321) construction
  line L62 (-40.2957, 30.3321) -> (-26.2907, 30.3321) construction
  line L63 (-26.2907, 30.3321) -> (-26.2907, 16.3271) construction
  line L64 (-26.2907, 16.3271) -> (-40.2957, 16.3271) construction
  line L65 (-40.2957, 16.3271) -> (-40.2957, 30.3321) construction
  line L66 (-21.2457, 30.3321) -> (-7.2407, 30.3321) construction
  line L67 (-7.2407, 30.3321) -> (-7.2407, 16.3271) construction
  line L68 (-7.2407, 16.3271) -> (-21.2457, 16.3271) construction
  line L69 (-21.2457, 16.3271) -> (-21.2457, 30.3321) construction
  line L70 (-2.1957, 30.3321) -> (11.8093, 30.3321) construction
  line L71 (11.8093, 30.3321) -> (11.8093, 16.3271) construction
  line L72 (11.8093, 16.3271) -> (-2.1957, 16.3271) construction
  line L73 (-2.1957, 16.3271) -> (-2.1957, 30.3321) construction
  line L74 (-11.8477, 11.2821) -> (2.1573, 11.2821) construction
  line L75 (2.1573, 11.2821) -> (2.1573, -2.7229) construction
  line L76 (2.1573, -2.7229) -> (-11.8477, -2.7229) construction
  line L77 (-11.8477, -2.7229) -> (-11.8477, 11.2821) construction
  line L78 (-30.8977, 11.2821) -> (-16.8927, 11.2821) construction
  line L79 (-16.8927, 11.2821) -> (-16.8927, -2.7229) construction
  line L80 (-16.8927, -2.7229) -> (-30.8977, -2.7229) construction
  line L81 (-30.8977, -2.7229) -> (-30.8977, 11.2821) construction
  line L82 (-49.9477, 11.2821) -> (-35.9427, 11.2821) construction
  line L83 (-35.9427, 11.2821) -> (-35.9427, -2.7229) construction
  line L84 (-35.9427, -2.7229) -> (-49.9477, -2.7229) construction
  line L85 (-49.9477, -2.7229) -> (-49.9477, 11.2821) construction
  line L86 (-68.9977, 11.2821) -> (-54.9927, 11.2821) construction
  line L87 (-54.9927, 11.2821) -> (-54.9927, -2.7229) construction
  line L88 (-54.9927, -2.7229) -> (-68.9977, -2.7229) construction
  line L89 (-68.9977, -2.7229) -> (-68.9977, 11.2821) construction
  line L90 (-88.0477, 11.2821) -> (-74.0427, 11.2821) construction
  line L91 (-74.0427, 11.2821) -> (-74.0427, -2.7229) construction
  line L92 (-74.0427, -2.7229) -> (-88.0477, -2.7229) construction
  line L93 (-88.0477, -2.7229) -> (-88.0477, 11.2821) construction
  line L94 (-107.0977, 11.2033) -> (-93.0927, 11.2033) construction
  line L95 (-93.0927, 11.2033) -> (-93.0927, -2.8017) construction
  line L96 (-93.0927, -2.8017) -> (-107.0977, -2.8017) construction
  line L97 (-107.0977, -2.8017) -> (-107.0977, 11.2033) construction
  line L98 (-112.1427, 11.2821) -> (-112.1427, -2.7229) construction
  line L99 (-112.1427, -2.7229) -> (-126.1477, -2.7229) construction
  line L100 (-126.1477, -2.7229) -> (-126.1477, 11.2821) construction
  line L101 (-126.1477, 11.2821) -> (-112.1427, 11.2821) construction
  line L102 (-145.1977, 11.2821) -> (-131.1927, 11.2821) construction
  line L103 (-131.1927, 11.2821) -> (-131.1927, -2.7229) construction
  line L104 (-131.1927, -2.7229) -> (-145.1977, -2.7229) construction
  line L105 (-145.1977, -2.7229) -> (-145.1977, 11.2821) construction
  line L106 (-164.2477, 11.2821) -> (-150.2427, 11.2821) construction
  line L107 (-150.2427, 11.2821) -> (-150.2427, -2.7229) construction
  line L108 (-150.2427, -2.7229) -> (-164.2477, -2.7229) construction
  line L109 (-164.2477, -2.7229) -> (-164.2477, 11.2821) construction
  line L110 (-183.2977, 11.2821) -> (-169.2927, 11.2821) construction
  line L111 (-169.2927, 11.2821) -> (-169.2927, -2.7229) construction
  line L112 (-169.2927, -2.7229) -> (-183.2977, -2.7229) construction
  line L113 (-183.2977, -2.7229) -> (-183.2977, 11.2821) construction
  line L114 (-211.7457, 11.2821) -> (-197.7407, 11.2821) construction
  line L115 (-197.7407, 11.2821) -> (-197.7407, -2.7229) construction
  line L116 (-197.7407, -2.7229) -> (-211.7457, -2.7229) construction
  line L117 (-211.7457, -2.7229) -> (-211.7457, 11.2821) construction
  line L118 (-197.5217, -7.7679) -> (-183.5167, -7.7679) construction
  line L119 (-183.5167, -7.7679) -> (-183.5167, -21.7729) construction
  line L120 (-183.5167, -21.7729) -> (-197.5217, -21.7729) construction
  line L121 (-197.5217, -21.7729) -> (-197.5217, -7.7679) construction
  line L122 (-178.4717, -7.7679) -> (-164.4667, -7.7679) construction
  line L123 (-164.4667, -7.7679) -> (-164.4667, -21.7729) construction
  line L124 (-164.4667, -21.7729) -> (-178.4717, -21.7729) construction
  line L125 (-178.4717, -21.7729) -> (-178.4717, -7.7679) construction
  line L126 (-159.4217, -7.7679) -> (-145.4167, -7.7679) construction
  line L127 (-145.4167, -7.7679) -> (-145.4167, -21.7729) construction
  line L128 (-145.4167, -21.7729) -> (-159.4217, -21.7729) construction
  line L129 (-159.4217, -21.7729) -> (-159.4217, -7.7679) construction
  line L130 (-140.3717, -7.7679) -> (-126.3667, -7.7679) construction
  line L131 (-126.3667, -7.7679) -> (-126.3667, -21.7729) construction
  line L132 (-126.3667, -21.7729) -> (-140.3717, -21.7729) construction
  line L133 (-140.3717, -21.7729) -> (-140.3717, -7.7679) construction
  line L134 (-121.3217, -7.7679) -> (-107.3167, -7.7679) construction
  line L135 (-107.3167, -7.7679) -> (-107.3167, -21.7729) construction
  line L136 (-107.3167, -21.7729) -> (-121.3217, -21.7729) construction
  line L137 (-121.3217, -21.7729) -> (-121.3217, -7.7679) construction
  line L138 (-102.2717, -7.7679) -> (-88.2667, -7.7679) construction
  line L139 (-88.2667, -7.7679) -> (-88.2667, -21.7729) construction
  line L140 (-88.2667, -21.7729) -> (-102.2717, -21.7729) construction
  line L141 (-102.2717, -21.7729) -> (-102.2717, -7.7679) construction
  line L142 (-83.2217, -7.7679) -> (-69.2167, -7.7679) construction
  line L143 (-69.2167, -7.7679) -> (-69.2167, -21.7729) construction
  line L144 (-69.2167, -21.7729) -> (-83.2217, -21.7729) construction
  line L145 (-83.2217, -21.7729) -> (-83.2217, -7.7679) construction
  line L146 (-64.1717, -7.7679) -> (-50.1667, -7.7679) construction
  line L147 (-50.1667, -7.7679) -> (-50.1667, -21.7729) construction
  line L148 (-50.1667, -21.7729) -> (-64.1717, -21.7729) construction
  line L149 (-64.1717, -21.7729) -> (-64.1717, -7.7679) construction
  line L150 (-45.1217, -7.7679) -> (-31.1167, -7.7679) construction
  line L151 (-31.1167, -7.7679) -> (-31.1167, -21.7729) construction
  line L152 (-31.1167, -21.7729) -> (-45.1217, -21.7729) construction
  line L153 (-45.1217, -21.7729) -> (-45.1217, -7.7679) construction
  line L154 (-26.0717, -7.7679) -> (-12.0667, -7.7679) construction
  line L155 (-12.0667, -7.7679) -> (-12.0667, -21.7729) construction
  line L156 (-12.0667, -21.7729) -> (-26.0717, -21.7729) construction
  line L157 (-26.0717, -21.7729) -> (-26.0717, -7.7679) construction
  line L158 (-6.7677, -7.7679) -> (7.2373, -7.7679) construction
  line L159 (7.2373, -7.7679) -> (7.2373, -21.7729) construction
  line L160 (7.2373, -21.7729) -> (-6.7677, -21.7729) construction
  line L161 (-6.7677, -21.7729) -> (-6.7677, -7.7679) construction
  line L162 (-16.4257, -26.8399) -> (-2.4207, -26.8399) construction
  line L163 (-2.4207, -26.8399) -> (-2.4207, -40.8449) construction
  line L164 (-2.4207, -40.8449) -> (-16.4257, -40.8449) construction
  line L165 (-16.4257, -40.8449) -> (-16.4257, -26.8399) construction
  line L166 (-35.4757, -26.8399) -> (-21.4707, -26.8399) construction
  line L167 (-21.4707, -26.8399) -> (-21.4707, -40.8449) construction
  line L168 (-21.4707, -40.8449) -> (-35.4757, -40.8449) construction
  line L169 (-35.4757, -40.8449) -> (-35.4757, -26.8399) construction
  line L170 (-54.5197, -26.8179) -> (-40.5147, -26.8179) construction
  line L171 (-40.5147, -26.8179) -> (-40.5147, -40.8229) construction
  line L172 (-40.5147, -40.8229) -> (-54.5197, -40.8229) construction
  line L173 (-54.5197, -40.8229) -> (-54.5197, -26.8179) construction
  line L174 (-73.5697, -26.8179) -> (-59.5647, -26.8179) construction
  line L175 (-59.5647, -26.8179) -> (-59.5647, -40.8229) construction
  line L176 (-59.5647, -40.8229) -> (-73.5697, -40.8229) construction
  line L177 (-73.5697, -40.8229) -> (-73.5697, -26.8179) construction
  line L178 (-92.6197, -26.8179) -> (-78.6147, -26.8179) construction
  line L179 (-78.6147, -26.8179) -> (-78.6147, -40.8229) construction
  line L180 (-78.6147, -40.8229) -> (-92.6197, -40.8229) construction
  line L181 (-92.6197, -40.8229) -> (-92.6197, -26.8179) construction
  line L182 (-111.6697, -26.8179) -> (-97.6647, -26.8179) construction
  line L183 (-97.6647, -26.8179) -> (-97.6647, -40.8229) construction
  line L184 (-97.6647, -40.8229) -> (-111.6697, -40.8229) construction
  line L185 (-111.6697, -40.8229) -> (-111.6697, -26.8179) construction
  line L186 (-130.7197, -26.8179) -> (-116.7147, -26.8179) construction
  line L187 (-116.7147, -26.8179) -> (-116.7147, -40.8229) construction
  line L188 (-116.7147, -40.8229) -> (-130.7197, -40.8229) construction
  line L189 (-130.7197, -40.8229) -> (-130.7197, -26.8179) construction
  line L190 (-149.7697, -26.8179) -> (-135.7647, -26.8179) construction
  line L191 (-135.7647, -26.8179) -> (-135.7647, -40.8229) construction
  line L192 (-135.7647, -40.8229) -> (-149.7697, -40.8229) construction
  line L193 (-149.7697, -40.8229) -> (-149.7697, -26.8179) construction
  line L194 (-168.8197, -26.8179) -> (-154.8147, -26.8179) construction
  line L195 (-154.8147, -26.8179) -> (-154.8147, -40.8229) construction
  line L196 (-154.8147, -40.8229) -> (-168.8197, -40.8229) construction
  line L197 (-168.8197, -40.8229) -> (-168.8197, -26.8179) construction
  line L198 (-187.8697, -26.8179) -> (-173.8647, -26.8179) construction
  line L199 (-173.8647, -26.8179) -> (-173.8647, -40.8229) construction
  line L200 (-173.8647, -40.8229) -> (-187.8697, -40.8229) construction
  line L201 (-187.8697, -40.8229) -> (-187.8697, -26.8179) construction
  line L202 (-214.0317, -26.8179) -> (-200.0267, -26.8179) construction
  line L203 (-200.0267, -26.8179) -> (-200.0267, -40.8229) construction
  line L204 (-200.0267, -40.8229) -> (-214.0317, -40.8229) construction
  line L205 (-214.0317, -40.8229) -> (-214.0317, -26.8179) construction
  line L206 (-205.1417, -45.8679) -> (-191.1367, -45.8679) construction
  line L207 (-191.1367, -45.8679) -> (-191.1367, -59.8729) construction
  line L208 (-191.1367, -59.8729) -> (-205.1417, -59.8729) construction
  line L209 (-205.1417, -59.8729) -> (-205.1417, -45.8679) construction
  line L210 (-181.2657, -45.8679) -> (-167.2607, -45.8679) construction
  line L211 (-167.2607, -45.8679) -> (-167.2607, -59.8729) construction
  line L212 (-167.2607, -59.8729) -> (-181.2657, -59.8729) construction
  line L213 (-181.2657, -59.8729) -> (-181.2657, -45.8679) construction
  line L214 (-83.7297, -45.8679) -> (-69.7247, -45.8679) construction
  line L215 (-69.7247, -45.8679) -> (-69.7247, -59.8729) construction
  line L216 (-69.7247, -59.8729) -> (-83.7297, -59.8729) construction
  line L217 (-83.7297, -59.8729) -> (-83.7297, -45.8679) construction
  line L218 (-219.7432, 11.2821) -> (-213.7432, 11.2821) construction
  line L219 (-213.7432, 11.2821) -> (-213.7432, -1.1179) construction
  line L220 (-213.7432, -1.1179) -> (-219.7432, -1.1179) construction
  line L221 (-219.7432, -1.1179) -> (-219.7432, 11.2821) construction
  line L222 (-195.7432, 11.2821) -> (-189.7432, 11.2821) construction
  line L223 (-189.7432, 11.2821) -> (-189.7432, -1.1179) construction
  line L224 (-189.7432, -1.1179) -> (-195.7432, -1.1179) construction
  line L225 (-195.7432, -1.1179) -> (-195.7432, 11.2821) construction
  line L226 (-12.9772, -45.8679) -> (-6.9772, -45.8679) projected
  line L227 (-10.9772, -45.8679) -> (-8.9772, -45.8679)
  line L228 (-8.9772, -45.8679) -> (-8.9772, -44.8679)
  line L229 (-8.9772, -44.8679) -> (-10.9772, -44.8679)
  line L230 (-10.9772, -44.8679) -> (-10.9772, -45.8679)
  line L231 (-144.4772, -45.8679) -> (-142.4772, -45.8679)
  line L232 (-142.4772, -45.8679) -> (-142.4772, -44.8679)
  line L233 (-142.4772, -44.8679) -> (-144.4772, -44.8679)
  line L234 (-144.4772, -44.8679) -> (-144.4772, -45.8679)
  line L235 (-217.7432, 11.2821) -> (-215.7432, 11.2821)
  line L236 (-215.7432, 11.2821) -> (-215.7432, 12.2821)
  line L237 (-215.7432, 12.2821) -> (-217.7432, 12.2821)
  line L238 (-217.7432, 12.2821) -> (-217.7432, 11.2821)
  line L239 (-193.7432, 11.2821) -> (-191.7432, 11.2821)
  line L240 (-191.7432, 11.2821) -> (-191.7432, 12.2821)
  line L241 (-191.7432, 12.2821) -> (-193.7432, 12.2821)
  line L242 (-193.7432, 12.2821) -> (-193.7432, 11.2821)
  point P0 (0, 0)
  point P1 (-9.9772, -45.8679)
  point P2 (-143.4772, -45.8679)
  point P3 (-216.7432, 11.2821)
  point P4 (-192.7432, 11.2821)
  dimension "d348" = 2
  dimension "d349" = 1
  dimension "d350" = 2
  dimension "d351" = 1
  dimension "d352" = 2
  dimension "d353" = 1
  dimension "d354" = 2
  dimension "d355" = 1
  constraints: 32 end point, 8 midpoint, 8 parallel, 4 horizontal, 4 perpendicular, 4 point on line
  measures "d348" distance of L229.end L228.end
  measures "d349" distance of L228.end L227.end
  measures "d350" distance of L233.end L232.end
  measures "d351" distance of L232.end L231.end
  measures "d352" distance of L237.end L236.end
  measures "d353" distance of L236.end L235.end
  measures "d354" distance of L241.end L240.end
  measures "d355" distance of L240.end L239.end
extrude "Extrusion10" cut sketch "Sketch9" against normal up to surface (3.25 mm away)
sketch "Sketch10" plane through (0, 0, 2) normal (0, 0, -1) x (-1, 0, 0)
  line L0 (12.9772, -48.3679) -> (12.9772, -45.8679) projected
  line L1 (6.9772, -42.3679) -> (146.4772, -42.3679) projected
  line L2 (12.9772, -48.3679) -> (140.4772, -48.3679)
  line L3 (140.4772, -48.3679) -> (140.4772, -42.3679)
  line L4 (140.4772, -42.3679) -> (12.9772, -42.3679)
  line L5 (12.9772, -42.3679) -> (12.9772, -48.3679)
  line L6 (140.4772, -45.8679) -> (140.4772, -48.3679) projected
  line L7 (195.7432, 8.7821) -> (195.7432, 11.2821) projected
  line L8 (189.7432, 14.7821) -> (219.7432, 14.7821) projected
  line L9 (195.7432, 8.7821) -> (213.7432, 8.7821)
  line L10 (213.7432, 8.7821) -> (213.7432, 14.7821)
  line L11 (213.7432, 14.7821) -> (195.7432, 14.7821)
  line L12 (195.7432, 14.7821) -> (195.7432, 8.7821)
  line L13 (213.7432, 11.2821) -> (213.7432, 8.7821) projected
  point P0 (0, 0)
  point P1 (12.9772, -42.3679)
  constraints: 16 end point, 4 parallel, 2 collinear, 2 horizontal, 2 perpendicular, 2 point on line
extrude "Extrusion11" cut sketch "Sketch10" against normal blind 0.5
equation "\"sw\" = 14.005"
equation "\"ipg\" = 0.1"
body "Solid5"
